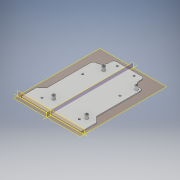
# Autodesk Inventor part: waveshare_expansion_board
Saved by Autodesk Inventor 2019 (Build 230136000, 136)
## iProperties
Created: 2021-05-27
Part Number: waveshare_expansion_board
Material: Generisch
Document SubType Name: Modeling
Designer: Lukas
Density: 1 g/cm^3
Appearance: Vorgabe
Author: Lukas
Autodesk Inventor part; units mm, degrees
sketch "Skizze1" plane through (0, 0, 0) normal (0, 1, 0) x (-1, 0, 0)
  line L0 (0, 0) -> (-52, 0)
  line L1 (-52, 0) -> (-52, -27)
  line L2 (-52, -27) -> (-42.5, -35.8741)
  line L3 (-42.5, -35.8741) -> (-42.5, -115.8741)
  line L4 (-42.5, -115.8741) -> (-26.5, -115.8741)
  line L5 (-26.5, -115.8741) -> (-26.5, -134.8741)
  line L6 (-26.5, -134.8741) -> (0, -134.8741)
  line L7 (0, -134.8741) -> (0, 0)
  dimension "d2" = 52
  dimension "d3" = 27
  dimension "d4" = 13
  dimension "d8" = 80
  dimension "d9" = 16
  dimension "d10" = 19
  dimension "d11" = 42.5
  dimension "d12" = 26.5
  dimension "d13" = 134.8741
  constraints: 16 end point, 3 perpendicular, 2 horizontal, 2 vertical
  measures "d2" distance of L0.start L0.end
  measures "d3" distance of L0.end L1.end
  measures "d4" distance of L1.end L2.end
  measures "d8" distance of L2.end L3.end
  measures "d9" distance of L3.end L4.end
  measures "d10" distance of L4.end L5.end
  measures "d11" horizontal distance of L0.start L2.end
  measures "d12" distance of L5.end L6.end
  measures "d13" distance of L6.end L0.start
extrude "Extrusion1" add sketch "Skizze1" along normal blind 1.5
fillet "Rundung1" radius 2 1 edges at (52, 0.75, 0)
fillet "Rundung2" radius 10 1 edges at (26.5, 0.75, -115.8741)
fillet "Rundung3" radius 5 1 edges at (42.5, 0.75, -115.8741)
fillet "Rundung4" radius 5 1 edges at (26.5, 0.75, -134.8741)
mirror "Spiegeln1" about plane through (0, 0, 0) normal (1, 0, 0) of "Extrusion1"
mirror "Spiegeln2" about plane through (0, 0, 0) normal (1, 0, 0) of "Rundung2", "Rundung4", "Rundung3", "Rundung1"
sketch "Skizze2" plane through (0, 1.5, 0) normal (0, 1, 0) x (1, 0, 0)
  line L0 (-26.5, 125.8741) -> (-26.5, 129.8741) projected
  line L1 (21.5, 134.8741) -> (-21.5, 134.8741) projected
  line L2 (26.5, 125.8741) -> (26.5, 129.8741) projected
  point P0 (0, 0)
  point P1 (14.5, 128.8741)
  point P2 (-14.5, 128.8741)
  dimension "d20" = 12
  dimension "d21" = 6
  dimension "d22" = 6
  dimension "d23" = 12
  measures "d20" distance from line of L0 point (-14.5, 128.874)
  measures "d21" distance from line of L1 point (-14.5, 128.874)
  measures "d22" distance from line of L1 point (14.5, 128.874)
  measures "d23" distance from line of L2 point (14.5, 128.874)
hole "Bohrung1" at (14.5, 1.5, -128.8741) at (-14.5, 1.5, -128.8741) direction (0, -1, 0) diameter 3 end through all
sketch "Skizze3" plane through (0, 1.5, 0) normal (0, 1, 0) x (1, 0, 0)
  line L0 (-52, 2) -> (-52, 27) projected
  line L1 (50, 0) -> (-50, 0) projected
  line L2 (52, 2) -> (52, 27) projected
  point P0 (0, 0)
  point P1 (32, 17)
  point P2 (-32, 17)
  point P3 (-32, 87)
  point P4 (32, 87)
  dimension "d31" = 20
  dimension "d32" = 17
  dimension "d33" = 20
  dimension "d34" = 17
  dimension "d42" = 70
  dimension "d43" = 70
  dimension "d44" = 20
  dimension "d45" = 20
  measures "d31" distance from line of point (-32, 17) L0
  measures "d32" distance from line of L1 point (-32, 17)
  measures "d33" distance from line of L2 point (32, 17)
  measures "d34" distance from line of L1 point (32, 17)
  measures "d42" distance of point (-32, 17) point (-32, 87)
  measures "d43" distance of point (32, 17) point (32, 87)
  measures "d44" distance from line of L2 point (32, 87)
  measures "d45" distance from line of L0 point (-32, 87)
hole "Bohrung3" at (32, 1.5, -17) at (-32, 1.5, -17) at (-32, 1.5, -87) at (32, 1.5, -87) direction (0, -1, 0) diameter 3 end through all
sketch "Skizze4" plane through (0, 1.5, 0) normal (0, 1, 0) x (1, 0, 0)
  circle A0 centre (37, 25) radius 2.5
  line L0 (50, 0) -> (-50, 0) projected
  line L1 (52, 2) -> (52, 27) projected
  circle A1 centre (37, 111) radius 2.5
  circle A2 centre (-20, 25) radius 2.5
  circle A3 centre (-20, 111) radius 2.5
  point P0 (0, 0)
  dimension "d53" = 5
  dimension "d54" = 25
  dimension "d55" = 15
  dimension "d56" = 5
  dimension "d57" = 86
  dimension "d58" = 15
  dimension "d59" = 5
  dimension "d60" = 25
  dimension "d61" = 57
  dimension "d62" = 5
  dimension "d63" = 57
  dimension "d64" = 86
  constraints: 4 centre point
  measures "d53" diameter of A0
  measures "d54" distance from line of L0 A0.centre
  measures "d55" distance from line of L1 A0.centre
  measures "d56" diameter of A1
  measures "d57" distance of A0.centre A1.centre
  measures "d58" distance from line of L1 A1.centre
  measures "d59" diameter of A2
  measures "d60" distance from line of L0 A2.centre
  measures "d61" distance of A0.centre A2.centre
  measures "d62" diameter of A3
  measures "d63" distance of A3.centre A1.centre
  measures "d64" distance of A2.centre A3.centre
extrude "Extrusion2" add sketch "Skizze4" along normal blind 6
sketch "Skizze5" plane through (-20, 7.5, -25) normal (0, 1, 0) x (1, 0, 0)
  circle A0 centre (57, 0) radius 2.5 projected
  circle A1 centre (57, 86) radius 2.5 projected
  circle A2 centre (0, 0) radius 2.5 projected
  circle A3 centre (0, 86) radius 2.5 projected
  point P0 (20, -25)
  dimension "d68" = 0
  dimension "d69" = 0
  dimension "d70" = 0
  dimension "d71" = 0
  dimension "d72" = 0
  dimension "d73" = 0
  dimension "d74" = 0
  dimension "d75" = 0
  measures "d68" distance of A1.centre point (57, 86)
  measures "d69" distance of A1.centre point (57, 86)
  measures "d70" distance of A0.centre point (57, 0)
  measures "d71" distance of A0.centre point (57, 0)
  measures "d72" distance of A2.centre point (0, 0)
  measures "d73" distance of A2.centre point (0, 0)
  measures "d74" distance of A3.centre point (0, 86)
  measures "d75" distance of A3.centre point (0, 86)
hole "Bohrung4" at (37, 7.5, -111) at (37, 7.5, -25) at (-20, 7.5, -25) at (-20, 7.5, -111) direction (0, -1, 0) diameter 3 end through all
thread "Gewinde1" size "M3x0.5" class "6H" standard "ANSI Metric M Profile" full length
thread "Gewinde2" size "M3x0.5" class "6H" standard "ANSI Metric M Profile" full length
thread "Gewinde3" size "M3x0.5" class "6H" standard "ANSI Metric M Profile" full length
thread "Gewinde4" size "M3x0.5" class "6H" standard "ANSI Metric M Profile" full length
ref_plane "Arbeitsebene1" through (0, 0, 0) normal (1, 0, 0) x (0, 1, 0)
